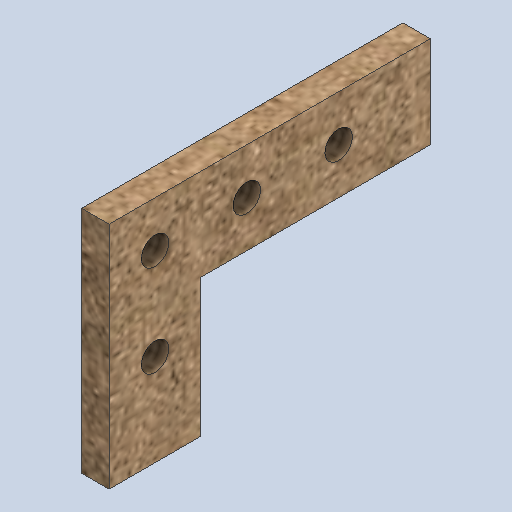
# Autodesk Inventor part: belt_liner_v1_MDF_F_1
Saved by Autodesk Inventor 2025.1 (Build 291241000, 241)
## iProperties
Created: 2024-12-15
Part Number: belt_liner_v1_MDF_F_1
Material: MDF 中密度繊維ボード
Document SubType Name: Modeling
Designer: haruy
Density: 0.8 g/cm^3
Appearance: ダンボール - 段ボール紙
Author: haruy
Autodesk Inventor part; units mm, degrees
ref_plane "YZ Plane" through (0, 0, 0) normal (1, 0, 0) x (0, 1, 0)
ref_plane "XZ Plane" through (0, 0, 0) normal (0, 1, 0) x (-1, 0, 0)
ref_plane "XY Plane" through (0, 0, 0) normal (0, 0, 1) x (1, 0, 0)
sketch "スケッチ1" plane through (0, 0, 0) normal (1, 0, 0) x (0, 1, 0)
  line L0 (-115.2146, 152.1685) -> (124.7854, 152.1685)
  line L1 (124.7854, 152.1685) -> (114.7854, 152.1685)
  line L2 (114.7854, 152.1685) -> (114.7854, -77.8315)
  line L3 (114.7854, -77.8315) -> (124.7854, -77.8315)
  line L4 (124.7854, -77.8315) -> (124.7854, 152.1685)
  line L5 (-115.2146, 152.1685) -> (-105.2146, 152.1685)
  line L6 (-105.2146, 152.1685) -> (-105.2146, -77.8315)
  line L7 (-105.2146, -77.8315) -> (-115.2146, -77.8315)
  line L8 (-115.2146, -77.8315) -> (-115.2146, 152.1685)
  line L9 (124.7854, 152.1685) -> (124.7854, 162.1685)
  line L10 (-115.2146, 162.1685) -> (124.7854, 162.1685)
  line L11 (4.7854, 162.1685) -> (4.7854, -110.7311)
  line L12 (124.7854, 127.1685) -> (114.7854, 127.1685)
  line L13 (99.7854, 152.1685) -> (99.7854, 162.1685)
  circle A0 centre (119.7854, 137.1685) radius 1.5
  circle A1 centre (119.7854, 147.1685) radius 1.5
  circle A2 centre (119.7854, 157.1685) radius 1.5
  circle A3 centre (109.7854, 157.1685) radius 1.5
  line L14 (114.7854, 152.1685) -> (99.7854, 152.1685)
  line L15 (124.7854, 152.1685) -> (124.7854, 162.1685)
  line L16 (124.7854, 162.1685) -> (99.7854, 162.1685)
  point P0 (0, 0)
  point P1 (4.7854, -147.8315)
  point P2 (-110.2146, 157.1685)
  point P3 (-100.2146, 157.1685)
  point P4 (-110.2146, 147.1685)
  point P5 (-110.2146, 137.1685)
  dimension "d0" = 10
  dimension "d1" = 230
  dimension "d2" = 10
  dimension "d3" = 230
  dimension "d4" = 5
  dimension "d5" = 10
  dimension "d6" = 5
  dimension "d7" = 5
  dimension "d8" = 5
  dimension "d9" = 10
  dimension "d10" = 5
  dimension "d11" = 5
  dimension "d12" = 10
  dimension "d13" = 10
  dimension "d14" = 3
  dimension "d15" = 3
  dimension "d16" = 3
  dimension "d17" = 3
  constraints: 34 end point, 5 perpendicular, 4 centre point, 4 coincident, 4 parallel, 4 point on line, 4 symmetric about line, 2 collinear, 2 horizontal, 1 midpoint, 1 vertical
  measures "d0" distance of L3.end L2.end
  measures "d1" distance of L2.end L1.end
  measures "d2" distance of L6.end L7.end
  measures "d3" distance of L5.end L6.end
  measures "d4" distance from line of point (119.785, 157.168) L9
  measures "d5" distance of point (109.785, 157.168) point (119.785, 157.168)
  measures "d6" distance from line of point (119.785, 157.168) L10
  measures "d7" distance from line of point (109.785, 157.168) L10
  measures "d8" distance from line of point (119.785, 147.168) L0
  measures "d9" distance of point (119.785, 137.168) point (119.785, 147.168)
  measures "d10" distance from line of point (119.785, 147.168) L4
  measures "d11" distance from line of point (119.785, 137.168) L4
  measures "d12" distance from line of L13 point (109.785, 157.168)
  measures "d13" distance from line of L12 point (119.785, 137.168)
  measures "d14" diameter of A0
  measures "d15" diameter of A1
  measures "d16" diameter of A2
  measures "d17" diameter of A3
extrude "押し出し1" add sketch "スケッチ1" against normal blind 3 contours L13 L10 L9 L0 | L0 L4 L12 L2
equation "\"d7\" = d6"
equation "\"d11\" = d10"
